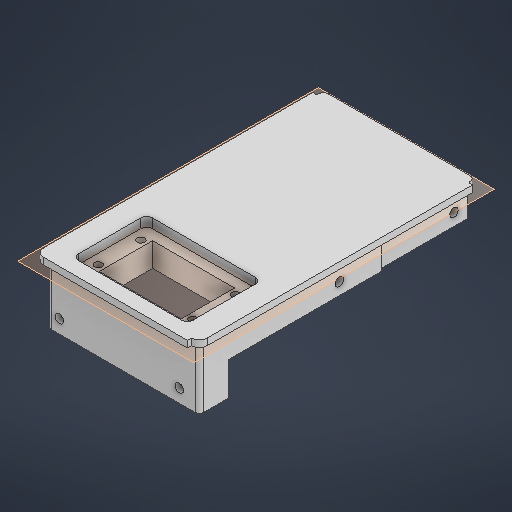
# Autodesk Inventor part: Endstueck_Harting
Saved by Autodesk Inventor 2026.1 (Build 301233020, 233B)
## iProperties
Created: 2025-06-04
Part Number: Endstueck_Harting
Material: Generic
Document SubType Name: Modeling
Designer: peter
Density: 1 g/cm^3
Appearance: Default
Author: peter
Autodesk Inventor part; units mm, degrees
ref_plane "YZ Plane" through (0, 0, 0) normal (1, 0, 0) x (0, 1, 0)
sketch "Sketch1" plane through (0, 0, 0) normal (0, 0, 1) x (1, 0, 0)
  line L0 (-137, -169) -> (-137, 30) projected
  line L1 (-140, 30) -> (-137, 30) projected
  line L2 (-140, 30) -> (-140, -169) projected
  arc A0 (-140, -169) -> (-134, -175) centre (-134, -169) ccw projected
  arc A1 (-137, -169) -> (-134, -172) centre (-134, -169) ccw projected
  line L3 (-134, -175) -> (-26, -175) projected
  line L4 (-26, -172) -> (-26, -175) projected
  line L5 (-26, -172) -> (-134, -172) projected
  line L6 (-26, -172) -> (-26, -175) projected
  arc A2 (-26, -175) -> (-20, -169) centre (-26, -169) ccw projected
  line L7 (-23, -169) -> (-20, -169) projected
  arc A3 (-26, -172) -> (-23, -169) centre (-26, -169) ccw projected
  line L8 (-23, -169) -> (-20, -169) projected
  line L9 (-20, -169) -> (-20, 30) projected
  line L10 (-20, 30) -> (-23, 30) projected
  line L11 (-23, 30) -> (-23, -169) projected
  line L12 (-137, 30) -> (-23, 30)
  line L13 (-137, -169) -> (-140, -169) projected
  line L14 (-140, -169) -> (-137, -169) projected
  line L15 (-134, -175) -> (-134, -172) projected
  line L16 (-134, -175) -> (-134, -172) projected
  constraints: 2 end point, 1 horizontal
extrude "Extrusion1" add sketch "Sketch1" against normal blind 20 contours L0 L12 L11 A3 L5 A1
sketch "Sketch2" plane through (0, 0, 0) normal (0, 0, 1) x (1, 0, 0)
  line L0 (-137, 30) -> (-23, 30) projected
  line L1 (-80, 30) -> (-80, -172) construction
  line L2 (-26, -172) -> (-134, -172) projected
  line L3 (-123, -167.1) -> (-37, -167.1)
  line L4 (-37, -167.1) -> (-37, -111.6)
  line L5 (-37, -111.6) -> (-123, -111.6)
  line L6 (-123, -111.6) -> (-123, -167.1)
  line L7 (-123, -167.1) -> (-37, -111.6) construction
  line L8 (-37, -167.1) -> (-123, -111.6) construction
  point P0 (0, 0)
  point P1 (-80, -139.35)
  dimension "d2" = 86
  dimension "d3" = 55.5
  dimension "d4" = 4.9
  constraints: 14 end point, 4 midpoint, 2 parallel, 1 horizontal, 1 perpendicular, 1 point on line
  measures "d2" distance of L5.end L4.end
  measures "d3" distance of L4.end L3.end
  measures "d4" distance between parallel lines of L2 L3
extrude "Extrusion2" cut sketch "Sketch2" against normal blind 2
sketch "Sketch3" plane through (0, 0, -2) normal (0, 0, 1) x (1, 0, 0)
  line L0 (-80, 30) -> (-80, -172) construction
  line L1 (-49.25, -159.35) -> (-110.75, -159.35)
  line L2 (-110.75, -159.35) -> (-110.75, -119.35)
  line L3 (-110.75, -119.35) -> (-49.25, -119.35)
  line L4 (-49.25, -119.35) -> (-49.25, -159.35)
  line L5 (-49.25, -159.35) -> (-110.75, -119.35) construction
  line L6 (-110.75, -159.35) -> (-49.25, -119.35) construction
  line L7 (-44.5, -155.35) -> (-115.5, -155.35) construction
  line L8 (-115.5, -155.35) -> (-115.5, -123.35) construction
  line L9 (-115.5, -123.35) -> (-44.5, -123.35) construction
  line L10 (-44.5, -123.35) -> (-44.5, -155.35) construction
  line L11 (-44.5, -155.35) -> (-115.5, -123.35) construction
  line L12 (-115.5, -155.35) -> (-44.5, -123.35) construction
  point P0 (0, 0)
  point P1 (-80, -139.35)
  dimension "d7" = 61.5
  dimension "d8" = 40
  dimension "d9" = 71
  dimension "d10" = 32
  constraints: 24 end point, 4 coincident, 4 midpoint, 4 parallel, 2 horizontal, 2 perpendicular
  measures "d7" distance of L2.end L3.end
  measures "d8" distance of L1.end L2.end
  measures "d9" distance of L8.end L9.end
  measures "d10" distance of L7.end L8.end
extrude "Extrusion3" cut sketch "Sketch3" against normal through all
hole "Hole1" at (-115.5, -123.35, -2) at (-115.5, -155.35, -2) at (-44.5, -155.35, -2) at (-44.5, -123.35, -2) direction (0, 0, -1) diameter 5.7 end through all
fillet "Fillet1" radius 4.5 4 edges at (-37, -111.6, -1) (-37, -167.1, -1) (-123, -167.1, -1) (-123, -111.6, -1)
sketch "Sketch4" plane through (0, 0, 0) normal (0, 0, 1) x (1, 0, 0)
  arc A0 (-123, -162.6) -> (-118.5, -167.1) centre (-118.5, -162.6) ccw projected
  line L0 (-118.5, -167.1) -> (-41.5, -167.1) projected
  arc A1 (-41.5, -167.1) -> (-37, -162.6) centre (-41.5, -162.6) ccw projected
  line L1 (-37, -162.6) -> (-37, -116.1) projected
  arc A2 (-37, -116.1) -> (-41.5, -111.6) centre (-41.5, -116.1) ccw projected
  line L2 (-41.5, -111.6) -> (-118.5, -111.6) projected
  arc A3 (-118.5, -111.6) -> (-123, -116.1) centre (-118.5, -116.1) ccw projected
  line L3 (-123, -116.1) -> (-123, -162.6) projected
  line L4 (-26, -172) -> (-134, -172) projected
  arc A4 (-137, -169) -> (-134, -172) centre (-134, -169) ccw projected
  line L5 (-137, -169) -> (-137, 30) projected
  line L6 (-137, 30) -> (-23, 30) projected
  line L7 (-23, 30) -> (-23, -169) projected
  arc A5 (-26, -172) -> (-23, -169) centre (-26, -169) ccw projected
  line L8 (-140, -169) -> (-140, 30)
  line L9 (-140, 30) -> (-137, 30)
  line L10 (-137, 30) -> (-137, -169)
  arc A6 (-137, -169) -> (-134, -172) centre (-134, -169) ccw
  line L11 (-134, -172) -> (-26, -172)
  arc A7 (-26, -172) -> (-23, -169) centre (-26, -169) ccw
  line L12 (-23, -169) -> (-23, 30)
  line L13 (-23, 30) -> (-20, 30)
  line L14 (-20, 30) -> (-20, -169)
  arc A8 (-26, -175) -> (-20, -169) centre (-26, -169) ccw
  line L15 (-26, -175) -> (-134, -175)
  arc A9 (-140, -169) -> (-134, -175) centre (-134, -169) ccw
  point P0 (0, 0)
  constraints: 16 end point, 8 point on circle, 4 centre point, 4 horizontal, 4 vertical, 14 other
extrude "Extrusion4" add sketch "Sketch4" along normal blind 5
ref_plane "Work Plane1" through (0, 0, 0) normal (0, 0, 1) x (1, 0, 0)
sketch "Sketch5" plane through (0, 0, 0) normal (0, 0, 1) x (1, 0, 0)
  arc A0 (-133, 33) -> (-135, 31) centre (-133, 31) ccw projected
  line L0 (-135, -35) -> (-135, 31) projected
  line L1 (-20, 33) -> (-23, 33) projected
  arc A1 (-25, 31) -> (-27, 33) centre (-27, 31) ccw projected
  line L2 (-25, 31) -> (-25, -35) projected
  line L3 (-20, 33) -> (-23, 33) projected
  line L4 (-20, 30) -> (-140, 30) projected
  line L5 (-133, 33) -> (-27, 33)
  point P0 (0, 0)
  point P1 (-135, 30)
  point P2 (-25, 30)
  constraints: 2 end point, 1 horizontal
extrude "Extrusion5" add sketch "Sketch5" against normal blind 54
sketch "Sketch6" plane through (0, 0, 0) normal (0, 0, 1) x (1, 0, 0)
  line L0 (-27, 35) -> (-50, 35)
  arc A0 (-23, 31) -> (-27, 35) centre (-27, 31) ccw
  line L1 (-23, -35) -> (-23, 31)
  line L2 (-50, 35) -> (-54.5, 35)
  line L3 (-137, 31) -> (-137, -35)
  arc A1 (-133, 35) -> (-137, 31) centre (-133, 31) ccw
  line L4 (-110, 35) -> (-133, 35)
  line L5 (-110, 35) -> (-54.5, 35)
  line L6 (-20, 30) -> (-140, 30)
  line L7 (-25, 30) -> (-23, 30)
  line L8 (-137, 30) -> (-23, 30)
  point P0 (0, 0)
  point P1 (-23, 30)
extrude "Extrusion6" add sketch "Sketch6" along normal up to surface (5 mm away)
sketch "Sketch7" plane through (-133, 33, -54) normal (0, 1, 0) x (1, 0, 0)
  line L0 (23, 62) -> (23, -54) projected
  line L1 (83, -54) -> (83, 62) projected
  line L2 (106, -54) -> (0, -54) projected
  line L3 (106, -54) -> (106, 0) projected
  line L4 (0, 0) -> (106, 0) projected
  line L5 (0, -54) -> (0, 0) projected
  point P0 (133, -54)
  point P1 (83, 0)
  point P2 (23, 0)
  point P3 (23, -54)
ref_plane "Work Plane2" through (-133, 35, -790) normal (0, 1, 0) x (0, 0, 1)
extrude "Extrusion7" add sketch "Sketch7" along normal up to surface (2 mm away) contours L4 L1 L2 L0
sketch "Sketch8" plane through (0, 0, 5) normal (0, 0, 1) x (1, 0, 0)
  line L0 (-140, -172) -> (-140, 30) projected
  arc A0 (-140, -172) -> (-134, -178) centre (-134, -172) ccw projected
  line L1 (-134, -178) -> (28, -178) projected
  line L2 (-26, -175) -> (-26, -178) projected
  line L3 (-134, -175) -> (-26, -175) projected
  line L4 (-140, -167.4228) -> (-134, -175)
  point P0 (0, 0)
  constraints: 2 end point, 1 point on line
ref_plane "Work Plane3" through (-134, -178, 0) normal (0, 0, 1) x (1, 0, 0)
extrude "Extrusion8" add sketch "Sketch8" against normal up to surface (5 mm away)
sketch "Sketch9" plane through (-23, -169, -20) normal (1, 0, 0) x (0, 0, -1)
  circle A0 centre (715, 169) radius 2.5 projected
  line L0 (660, 136) -> (770, 136) projected
  line L1 (770, 200) -> (770, 136) projected
  line L2 (-20, 200) -> (770, 200) projected
  line L3 (-20, 134) -> (-20, 200) projected
  line L4 (-20, 134) -> (0, 134) projected
  line L5 (0, 134) -> (660, 134) projected
  line L6 (660, 134) -> (660, 136) projected
  circle A1 centre (250, 190) radius 2.5 projected
  circle A2 centre (545, 190) radius 2.5 projected
  line L7 (-20, 200) -> (0, 200)
  line L8 (0, 200) -> (0, 134)
  line L9 (0, 134) -> (-20, 134)
  line L10 (-20, 134) -> (-20, 200)
  point P0 (-20, 169)
  constraints: 8 end point, 2 parallel, 1 horizontal, 1 perpendicular
extrude "Extrusion9" cut sketch "Sketch9" against normal blind 2 contours L4 L3 L2 L8
sketch "Sketch10" plane through (-137, -169, -20) normal (-1, 0, 0) x (0, 0, 1)
  line L0 (0, 199) -> (-34, 199) projected
  line L1 (-34, 200) -> (-34, 199) projected
  line L2 (20, 200) -> (-34, 200) projected
  line L3 (20, 134) -> (20, 200) projected
  line L4 (0, 134) -> (20, 134) projected
  line L5 (0, 199) -> (0, 134) projected
  line L6 (20, 200) -> (0, 200)
  line L7 (0, 200) -> (0, 134)
  line L8 (0, 134) -> (20, 134)
  line L9 (20, 134) -> (20, 200)
  point P0 (20, 169)
  constraints: 8 end point, 2 parallel, 1 horizontal, 1 perpendicular
extrude "Extrusion10" cut sketch "Sketch10" against normal blind 2 contours L7 L2 L3 L4 L5
thicken "Thicken1" operation add thickness 3 both sides no extend neighbours no toward (0, -1, 0) faces at (-98.3333, 30, -31.3333)
chamfer "Chamfer2" distance 10.75 distance2 34 1 edges at (-80, 27, -20) measured on face at (-80, 26.5, -20)
sketch "Sketch11" plane through (0, 0, -20) normal (0, 0, -1) x (-1, 0, 0)
  line L0 (92.1988, -20.2227) -> (127.1988, -20.2227)
  line L1 (127.1988, -20.2227) -> (127.1988, -55.2227)
  line L2 (127.1988, -55.2227) -> (92.1988, -55.2227)
  line L3 (92.1988, -55.2227) -> (92.1988, -20.2227)
  line L4 (110, 35) -> (50, 35) projected
  line L5 (80, 35) -> (80, -42.8692) construction
  point P0 (0, 0)
  dimension "d44" = 35
  dimension "d45" = 35
  constraints: 10 end point, 2 parallel, 1 horizontal, 1 midpoint, 1 perpendicular, 1 vertical
  measures "d44" distance between parallel lines of L1 L3
  measures "d45" distance between parallel lines of L2 L0
extrude "Extrusion11" cut sketch "Sketch11" against normal blind 10
chamfer "Chamfer3" distance 5 angle 45 2 edges at (-109.6988, -20.2227, -20) (-109.6988, -55.2227, -20)
sketch "Sketch12" plane through (-137, -169, -20) normal (-1, 0, 0) x (0, 0, 1)
  circle A0 centre (9, 102) radius 3.2
  line L0 (25, 199) -> (25, -3) projected
  line L1 (20, 202) -> (-34, 202) projected
  point P0 (20, 169)
  dimension "d51" = 6.4
  dimension "d52" = 16
  dimension "d53" = 100
  constraints: 1 centre point
  measures "d51" diameter of A0
  measures "d52" distance from line of L0 A0.centre
  measures "d53" distance from line of L1 A0.centre
extrude "Extrusion12" cut sketch "Sketch12" against normal through all
sketch "Sketch13" plane through (-25, 31, 0) normal (1, 0, 0) x (0, 0, -1)
  circle A0 centre (270.0162, -10) radius 2.5 projected
  circle A1 centre (11, -10) radius 3.2
  circle A2 centre (11, -98) radius 3.2 projected
  point P0 (0, -31)
  dimension "d56" = 6.4
  constraints: 1 centre point, 1 horizontal alignment, 1 vertical alignment
  measures "d56" diameter of A1
extrude "Extrusion13" cut sketch "Sketch13" against normal through all contours A1
sketch "Sketch15" plane through (-27, 33, 0) normal (0, 1, 0) x (1, 0, 0)
  circle A0 centre (-95, 15) radius 2.8
  circle A1 centre (-11, 15) radius 2.8
  line L0 (-91.5, -5) -> (-14.5, -5) projected
  line L1 (-53, -5) -> (-53, 54) construction
  line L2 (2, 54) -> (-108, 54) projected
  line L3 (0, 0) -> (-106, 0) projected
  line L4 (-83, 0) -> (-83, 54) projected
  point P0 (27, 0)
  dimension "d64" = 5.6
  dimension "d65" = 15
  dimension "d66" = 12
  constraints: 2 centre point, 2 end point, 2 midpoint, 1 equal radius, 1 horizontal alignment, 1 symmetric about line
  measures "d64" diameter of A0
  measures "d65" distance from line of L3 A0.centre
  measures "d66" distance from line of L4 A0.centre
extrude "Extrusion15" cut sketch "Sketch15" against normal blind 12
sketch "Skizze16" plane through (-133, 35, 5) normal (0, 1, 0) x (1, 0, 0)
  line L0 (108, 25) -> (-2, 25) construction
  line L1 (0, 0) -> (106, 0) construction
  line L2 (106, 5) -> (106, 0) construction
  line L3 (23, 5) -> (0, 5) construction
  line L4 (83, 59) -> (83, 5) construction
  line L5 (23, 59) -> (83, 59) construction
  line L6 (23, 5) -> (23, 59) construction
  line L7 (106, 5) -> (83, 5) construction
  line L8 (0, 5) -> (0, 0) construction
  circle A0 centre (53, 44) radius 3.65
  point P0 (133, 5)
  point P1 (53, 59)
  dimension "d69" = 7.3
  dimension "d70" = 15
  constraints: 1 centre point, 1 midpoint, 1 vertical alignment
  measures "d69" diameter of A0
  measures "d70" distance from line of A0.centre L5
extrude "Extrusion16" cut sketch "Skizze16" against normal blind 21.75
sketch "Sketch17" plane through (0, 0, -20) normal (0, 0, -1) x (-1, 0, 0)
  line L0 (92.1988, -60.2227) -> (92.1988, -15.2227) projected
  line L1 (127.1988, -15.2227) -> (92.1988, -15.2227) projected
  line L2 (127.1988, -15.2227) -> (127.1988, -60.2227) projected
  line L3 (92.1988, -60.2227) -> (127.1988, -60.2227) projected
  line L4 (25, 16.25) -> (135, 16.25) projected
  line L5 (25, 16.25) -> (25, -35) projected
  line L6 (25, -35) -> (23, -35) projected
  line L7 (23, -35) -> (23, -169) projected
  arc A0 (23, -169) -> (26, -172) centre (26, -169) ccw projected
  line L8 (26, -172) -> (134, -172) projected
  arc A1 (134, -172) -> (137, -169) centre (134, -169) ccw projected
  line L9 (137, -169) -> (137, -35) projected
  line L10 (137, -35) -> (135, -35) projected
  line L11 (135, -35) -> (135, 16.25) projected
  circle A2 centre (44.5, -123.35) radius 2.85 projected
  circle A3 centre (44.5, -155.35) radius 2.85 projected
  circle A4 centre (115.5, -155.35) radius 2.85 projected
  circle A5 centre (115.5, -123.35) radius 2.85 projected
  line L12 (110.75, -119.35) -> (110.75, -159.35) projected
  line L13 (110.75, -159.35) -> (49.25, -159.35) projected
  line L14 (49.25, -159.35) -> (49.25, -119.35) projected
  line L15 (49.25, -119.35) -> (110.75, -119.35) projected
  line L16 (23, -164) -> (137, -164)
  line L17 (38, -164) -> (23, -149)
  line L18 (23, -35) -> (23, -169) projected
  line L19 (38, -164) -> (59.2132, -164) construction
  line L20 (26, -172) -> (134, -172) projected
  line L21 (80, -172) -> (80, -164) construction
  line L22 (122, -164) -> (137, -149)
  point P0 (0, 0)
  dimension "d73" = 8
  dimension "d74" = 135
  dimension "d75" = 15
  constraints: 10 end point, 4 point on line, 2 horizontal, 2 midpoint, 2 symmetric about line, 1 equal length
  measures "d73" distance between parallel lines of L8 L16
  measures "d74" angle of L19 L17
  measures "d75" distance of L16.start L17.start
extrude "Extrusion17" add sketch "Sketch17" along normal blind 25 contours L17 L16 L7 | L9 L16 L22 | L16 L9 A1 L8 A0 L7
chamfer "Chamfer4" distance 1 angle 45 1 edges at (-23, -149, -32.5)
chamfer "Chamfer5" distance 1 angle 45 1 edges at (-137, -149, -32.5)
sketch "Sketch18" plane through (-134, -172, 0) normal (0, -1, 0) x (1, 0, 0)
  circle A0 centre (96, -35) radius 3 construction
  circle A1 centre (6, -35) radius 3 construction
  circle A2 centre (96, -35) radius 3.2
  circle A3 centre (6, -35) radius 3.2
  point P0 (134, 0)
  dimension "d84" = 6.4
  dimension "d85" = 6.4
  constraints: 2 centre point, 2 coincident
  measures "d84" diameter of A2
  measures "d85" diameter of A3
extrude "Extrusion18" cut sketch "Sketch18" against normal blind 25
sketch "Skizze19" plane through (0, 0, -20) normal (0, 0, -1) x (-1, 0, 0)
  circle A0 centre (81.8514, 76.566) radius 96.3709
  point P0 (0, 0)
  constraints: 1 centre point
extrude "Extrusion19" cut sketch "Skizze19" along normal through all
body "Solid1"
